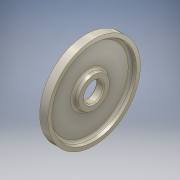
# Autodesk Inventor part: Wheel
Saved by Autodesk Inventor 2016 (Build 200138000, 138)
## iProperties
Created: 2021-04-07
Part Number: Wheel
Material: Типовые
Document SubType Name: Modeling
Designer: Лол
Density: 1 g/cm^3
Appearance: Титан
Author: Лол
Autodesk Inventor part; units mm, degrees
ref_plane "YZ Plane" through (0, 0, 0) normal (1, 0, 0) x (0, 1, 0)
ref_plane "XZ Plane" through (0, 0, 0) normal (0, 1, 0) x (-1, 0, 0)
ref_plane "XY Plane" through (0, 0, 0) normal (0, 0, 1) x (1, 0, 0)
sketch "Эскиз1" plane through (0, 0, 0) normal (0, 0, 1) x (1, 0, 0)
  line L0 (0, 17.5) -> (0, 28)
  line L1 (1, 28.2679) -> (1, 77.1486)
  line L2 (0, 77.4165) -> (0, 84.4165)
  line L3 (0, 84.4165) -> (15, 84.4165)
  line L4 (6, 75.005) -> (6, 30.4115)
  line L5 (15, 17.5) -> (0, 17.5)
  line L6 (15, 28) -> (15, 17.5)
  line L7 (-3, 0) -> (18, 0) construction
  line L8 (0, -16.8833) -> (0, 101.2998) construction
  line L9 (15, 84.4165) -> (15, 77.4165)
  line L10 (15, 77.4165) -> (6, 75.005)
  line L11 (15, 28) -> (6, 30.4115)
  line L12 (0, 28) -> (1, 28.2679)
  line L13 (0, 77.4165) -> (1, 77.1486)
  point P0 (0, 0)
  point P1 (1, 77.4165)
  point P2 (7, 77.4165)
  point P3 (7, 28)
  dimension "d0" = 15
  dimension "d2" = 5
  dimension "d5" = 35
  dimension "d7" = 168.833
  dimension "d9" = 0
  dimension "d17" = 75
  dimension "d18" = 75
  dimension "d19" = 56
  dimension "d20" = 75
  dimension "d21" = 75
  dimension "d22" = 2
  dimension "d24" = 7
  constraints: 24 end point, 4 parallel, 3 point on line, 2 perpendicular, 1 vertical
  measures "d0" distance of L2.end L3.end
  measures "d2" distance between parallel lines of L4 L1
  measures "d5" diameter of L5 L7
  measures "d7" diameter of L3 L7
  measures "d9" distance between parallel lines of L0 L8
  measures "d17" angle of L4 L10
  measures "d18" angle of L11 L4
  measures "d19" diameter of L6.start L7
  measures "d20" angle of L1 L13
  measures "d21" angle of L12 L1
  measures "d22" diameter of L1 L8
  measures "d24" distance from line of L3 L2.start
revolve "Вращение1" add sketch "Эскиз1" angle 360 about axis through (-10, 0, 0) along (1, 0, 0)
chamfer "Фаска1" distance 2 angle 45 2 edges at (15, -17.5, 0) (0, -17.5, 0)
fillet "Сопряжение3" radius 5 2 edges at (6, -75.005, 0) (6, -30.4115, 0)
fillet "Сопряжение4" radius 5 2 edges at (1, -28.2679, 0) (1, -77.1486, 0)
